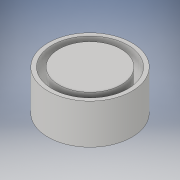
# Autodesk Inventor part: LargeFinderObjectiveCover
Saved by Autodesk Inventor 2019.1 (Build 231200000, 200)
## iProperties
Created: 2018-09-02
Part Number: LargeFinderObjectiveCover
Material: Generic
Document SubType Name: Modeling
Designer: steele
Density: 1 g/cm^3
Appearance: Default
Author: steele
Autodesk Inventor part; units mm, degrees
ref_plane "YZ Plane" through (0, 0, 0) normal (1, 0, 0) x (0, 1, 0)
ref_plane "XZ Plane" through (0, 0, 0) normal (0, 1, 0) x (-1, 0, 0)
ref_plane "XY Plane" through (0, 0, 0) normal (0, 0, 1) x (1, 0, 0)
sketch "Sketch1" plane through (0, 0, 0) normal (0, 1, 0) x (-1, 0, 0)
  circle A0 centre (0, 0) radius 33.32
  dimension "d0" = 66.64
  constraints: 1 centre point, 1 coincident
  measures "d0" diameter of A0
extrude "Extrusion1" add sketch "Sketch1" along normal blind 6.35
sketch "Sketch2" plane through (0, 6.35, 0) normal (0, 1, 0) x (1, 0, 0)
  circle A0 centre (0, 0) radius 33.32
  circle A1 centre (0, 0) radius 24.6825
  circle A2 centre (0, 0) radius 30.145
  dimension "d4" = 60.29
  dimension "d5" = 66.64
  dimension "d6" = 49.365
  constraints: 3 centre point, 3 coincident
  measures "d4" diameter of A2
  measures "d5" diameter of A0
  measures "d6" diameter of A1
extrude "Extrusion2" add sketch "Sketch2" along normal blind 25.4
equation "\"d0\" = lensCoverOD"
equation "\"d2\" = wallThickness"
equation "\"d4\" = objectiveOD"
equation "\"d5\" = lensCoverOD"
equation "\"d6\" = lensCoverID"
equation "\"d7\" = lensCoverLength"
equation "\"objectiveOD\" = 60.29"
equation "\"lensCoverLength\" = 25.4"
equation "\"wallThickness\" = 6.35"
equation "\"lensCoverOD\" = objectiveOD + wallThickness"
equation "\"printerClearance\" = 0.635"
equation "\"lensCoverID\" = objectiveID - printerClearance"
equation "\"objectiveID\" = 50"
body "Solid1"
